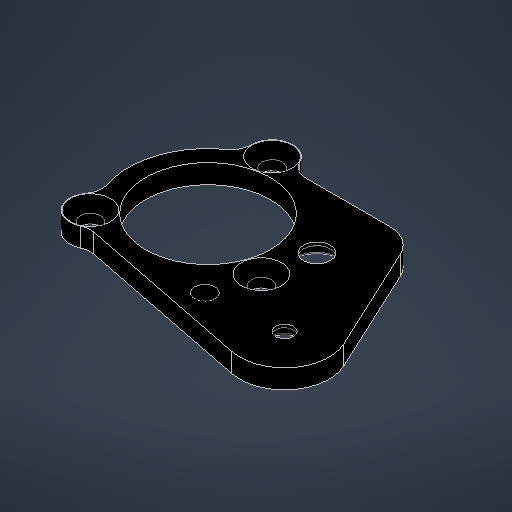
# Autodesk Inventor part: Dribbler Bracket A
Saved by Autodesk Inventor 2026.1 (Build 301233020, 233B)
## iProperties
Created: 2026-04-17
Part Number: Dribbler Bracket A
Material: Generic
Document SubType Name: Modeling
Designer: Bahaa
Mass: 1.71728 g
Surface Area: 20.4601 cm^2
Volume: 1.71728 cm^3
Density: 1 g/cm^3
Appearance: Default(1)
Author: Bahaa
Autodesk Inventor part; units mm, degrees
ref_plane "YZ Plane" through (0, 0, 0) normal (1, 0, 0) x (0, 1, 0)
ref_plane "XZ Plane" through (0, 0, 0) normal (0, 1, 0) x (-1, 0, 0)
ref_plane "XY Plane" through (0, 0, 0) normal (0, 0, 1) x (1, 0, 0)
sketch "Sketch1" plane through (0, 0, 0) normal (0, 0, 1) x (1, 0, 0)
  circle A0 centre (0, 0) radius 9.8
  circle A1 centre (0, 0) radius 12.5
  circle A2 centre (0, 0) radius 5 construction
  circle A3 centre (0, 0) radius 2.6
  circle A4 centre (22, -10) radius 6.25 construction
  circle A5 centre (13.8847, 3.2058) radius 9.25 construction
  circle A6 centre (22, -10) radius 7
  circle A7 centre (10.5, -11) radius 1.6
  circle A8 centre (10.5, -11) radius 3.75
  line L0 (-7.6147, -11.2266) -> (20.6297, -16.8646)
  line L1 (0, 12.5) -> (16.0464, 12.5)
  line L2 (20.5779, 9.6131) -> (28.3442, -7.0417)
  arc A9 (20.5779, 9.6131) -> (16.0464, 12.5) centre (16.0464, 7.5) ccw
  circle A10 centre (13.8847, 3.2058) radius 2.1
  circle A11 centre (13.8847, 3.2058) radius 3.5125
  circle A12 centre (13.8847, 3.2058) radius 4.1125
  circle A13 centre (22, -10) radius 1.4
  circle A14 centre (22, -10) radius 3.0125
  circle A15 centre (22, -10) radius 3.6125
  circle A16 centre (-9.698, -8.7322) radius 3.25
  circle A17 centre (-9.698, -8.7322) radius 1.6
  circle A18 centre (12.4113, -4.0327) radius 3.25
  circle A19 centre (12.4113, -4.0327) radius 1.6
  circle A20 centre (-2.7132, 12.7648) radius 3.25
  circle A21 centre (-2.7132, 12.7648) radius 1.6
  line L3 (0, 0) -> (-9.2893, -8.3641) construction
  line L4 (0, 0) -> (12.5, 0) construction
  arc A22 (10.1868, -12.569) -> (10.8132, -9.431) centre (10.5, -11) ccw
  point P0 (-2.4469, -12.2582)
  point P1 (0.5259, 12.5)
  point P2 (-5.5594, 11.1957)
  point P3 (-11.0783, -5.7898)
  point P4 (-6.9161, -10.4124)
  dimension "d33" = 6.5
  dimension "d0" = 19.6
  dimension "d1" = 25
  dimension "d2" = 10
  dimension "d3" = 5.2
  dimension "d4" = 22
  dimension "d5" = 10
  dimension "d6" = 12.5
  dimension "d7" = 18.5
  dimension "d8" = 14
  dimension "d9" = 3.2
  dimension "d10" = 11
  dimension "d11" = 10.5
  dimension "d12" = 7.5
  dimension "d13" = 115
  dimension "d14" = 5
  dimension "d15" = 4.2
  dimension "d16" = 7.025
  dimension "d17" = 8.225
  dimension "d18" = 2.8
  dimension "d19" = 6.025
  dimension "d20" = 7.225
  dimension "d34" = 3.2
  dimension "d37" = 360
  dimension "d39" = 12.5
  dimension "d40" = 138
  constraints: 22 centre point, 15 coincident, 10 end point, 8 point on circle, 8 tangent, 2 horizontal, 2 point on line, 1 equal length, 17 other
  measures "d0" diameter of A0
  measures "d1" diameter of A1
  measures "d2" diameter of A2
  measures "d3" diameter of A3
  measures "d4" horizontal distance of point (0, 0) A4.centre
  measures "d5" vertical distance of point (0, 0) A4.centre
  measures "d6" diameter of A4
  measures "d7" diameter of A5
  measures "d8" diameter of A6
  measures "d9" diameter of A7
  measures "d10" vertical distance of point (0, 0) A7.centre
  measures "d11" horizontal distance of point (0, 0) A7.centre
  measures "d12" diameter of A8
  measures "d13" angle of L2 L1
  measures "d14" radius of A9
  measures "d15" diameter of A10
  measures "d16" diameter of A11
  measures "d17" diameter of A12
  measures "d18" diameter of A13
  measures "d19" diameter of A14
  measures "d20" diameter of A15
  measures "d34" diameter of A17
  measures "d39" distance of L3.start L3.end
  measures "d40" angle of L3 L4
extrude "Extrusion1" add sketch "Sketch1" against normal blind 3 contours A0 A20 A1 A12 A18 | A0 A16 A1 A20 | A20 A1 A21 | A18 A1 A8 A16 A0 | A18 A1 A19 | A16 A1 A17 | A20 L1 A1 A21 | A20 L1 A9 L2 A6 L0 A1 A8 A18 A12 | A1 L1 A20 | A18 A1 A19 | A1 A17 A16 | A21 A1 | A1 A21 | A12 A1 A11 | A1 A11 A12 | A19 A1 | A1 A19 | A8 A1 | A1 A8 | A1 L0 A16 | A17 A1 | A1 A17 | A11 A1 A10 | A1 A10 A11 | A6 | A14 | A15
extrude "Extrusion2" cut sketch "Sketch1" along normal blind 0.6 from surface at -3 contours A12 A1 A11 | A1 A11 A12 | A15
extrude "Extrusion3" cut sketch "Sketch1" along normal blind 2.5 from surface at -3 contours A11 A1 A10 | A1 A10 A11 | A14
fillet "Fillet1" radius 3 4 edges at (-11.0783, -5.7898, -1.5) (-5.5594, 11.1957, -1.5) (0.5259, 12.5, -1.5) (-7.6147, -11.2266, -1.5)
hole "Hole1" at (-2.7132, 12.7648, 0) at (-9.698, -8.7322, 0) at (12.4113, -4.0327, 0) direction (0, 0, -1) diameter 3.2 depth 6 countersink diameter 6.3 countersink angle 90 clearance for "Countersunk Flat Head Screw DIN EN ISO 2009" size "M3" standard "DIN"
body "Solid1"
